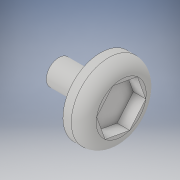
# Autodesk Inventor part: nit
Saved by Autodesk Inventor 2019 (Build 230136000, 136)
## iProperties
Created: 2020-01-12
Part Number: nit
Material: Ogólny
Document SubType Name: Modeling
Designer: Karolina
Density: 1 g/cm^3
Appearance: Domyślna
Author: Karolina
Autodesk Inventor part; units mm, degrees
ref_plane "YZ Plane" through (0, 0, 0) normal (1, 0, 0) x (0, 1, 0)
ref_plane "XZ Plane" through (0, 0, 0) normal (0, 1, 0) x (-1, 0, 0)
ref_plane "XY Plane" through (0, 0, 0) normal (0, 0, 1) x (1, 0, 0)
sketch "Szkic1" plane through (0, 0, 0) normal (0, 0, 1) x (1, 0, 0)
  line L0 (-0.3, 0) -> (1.8, 0) projected
  line L1 (0, -0.18) -> (0, 1.08) construction
  line L2 (0, 0) -> (0, 0.3)
  line L3 (0, 0.3) -> (1, 0.3)
  line L4 (1, 0.3) -> (1, 0.9)
  line L5 (1, 0.9) -> (1.5, 0.9)
  line L6 (1.5, 0.9) -> (1.5, 0)
  line L7 (0, 0) -> (1.5, 0)
  dimension "d0" = 0.3
  dimension "d1" = 1
  dimension "d2" = 0.6
  dimension "d3" = 0.5
  constraints: 12 end point, 3 perpendicular, 2 point on line, 1 collinear, 1 horizontal
  measures "d0" distance of L2.start L2.end
  measures "d1" distance of L2.end L3.end
  measures "d2" distance of L3.end L4.end
  measures "d3" distance of L4.end L5.end
revolve "Obrót1" add sketch "Szkic1" angle 360 about axis through (-10, 0, 0) along (1, 0, 0)
fillet "Zaokrąglenie1" radius 0.3 1 edges at (1.5, -0.9, 0)
sketch "Szkic2" plane through (1.5, 0, 0) normal (1, 0, 0) x (0, 0, -1)
  circle A0 centre (0, 0) radius 0.6 construction
  circle A1 centre (0, 0) radius 0.6 construction
  circle A2 centre (0, 0) radius 0.6 construction
  line L0 (0.2026, -0.5648) -> (-0.3878, -0.4578)
  line L1 (-0.3878, -0.4578) -> (-0.5904, 0.107)
  line L2 (-0.5904, 0.107) -> (-0.2026, 0.5648)
  line L3 (-0.2026, 0.5648) -> (0.3878, 0.4578)
  line L4 (0.3878, 0.4578) -> (0.5904, -0.107)
  line L5 (0.5904, -0.107) -> (0.2026, -0.5648)
  dimension "d6" = 0.4578
  constraints: 12 end point, 1 coincident, 15 other
  measures "d6" vertical distance of point (0, 0) L3.end
extrude "Wyciągnięcie proste1" cut sketch "Szkic2" against normal blind 0.3
